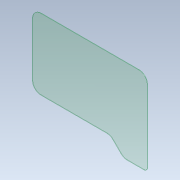
# Autodesk Inventor part: Стекло
Saved by Autodesk Inventor 2021.2 (Build 252289000, 289)
## iProperties
Created: 2022-11-29
Part Number: Стекло
Material: Типовые
Document SubType Name: ЛистМат
Designer: Voodoo
Density: 1 g/cm^3
Sheet Metal Rule: По умолчанию_мм
Appearance: Прозрачный — зеленый 1
Mass: 244.688 g
Surface Area: 2475.51 cm^2
Volume: 244.688 cm^3
Flat Pattern Width: 31.9 cm
Flat Pattern Length: 43.6 cm
Flat Pattern Area: 1390.84 cm^2
Sheet Metal Width: 319,000 мм
Sheet Metal Length: 436,000 мм
Sheet Metal Area: 139084,000 мм^2
Author: Voodoo
Autodesk Inventor part; units mm, degrees
ref_plane "YZ Plane" through (0, 0, 0) normal (1, 0, 0) x (0, 1, 0)
ref_plane "XZ Plane" through (0, 0, 0) normal (0, 1, 0) x (-1, 0, 0)
ref_plane "XY Plane" through (0, 0, 0) normal (0, 0, 1) x (1, 0, 0)
sketch "Эскиз1" plane through (0, 0, 0) normal (0, 0, 1) x (1, 0, 0)
  line L0 (-186, -134.5) -> (65.5736, -134.5)
  line L1 (218, -134.5) -> (218, 102.5)
  line L2 (186, 134.5) -> (-186, 134.5)
  line L3 (-218, 102.5) -> (-218, -102.5)
  line L4 (-218, -134.5) -> (218, 134.5) construction
  line L5 (218, -134.5) -> (-218, 134.5) construction
  arc A0 (-186, 134.5) -> (-218, 102.5) centre (-186, 102.5) ccw
  arc A1 (218, 102.5) -> (186, 134.5) centre (186, 102.5) ccw
  arc A2 (-218, -102.5) -> (-186, -134.5) centre (-186, -102.5) ccw
  line L6 (218, -134.5) -> (218, -172.5)
  line L7 (206, -184.5) -> (140.4264, -184.5)
  line L8 (119.2132, -175.7132) -> (86.7868, -143.2868)
  arc A3 (206, -184.5) -> (218, -172.5) centre (206, -172.5) ccw
  arc A4 (119.2132, -175.7132) -> (140.4264, -184.5) centre (140.4264, -154.5) ccw
  arc A5 (86.7868, -143.2868) -> (65.5736, -134.5) centre (65.5736, -164.5) ccw
  point P0 (0, 0)
  point P1 (218, -184.5)
  point P2 (128, -184.5)
  dimension "d2" = 436
  dimension "d3" = 269
  dimension "d4" = 32
  dimension "d5" = 319
  dimension "d6" = 12
  dimension "d7" = 50
  dimension "d8" = 90
  dimension "d9" = 135
  dimension "d10" = 30
  measures "d2" distance of L5.end L4.end
  measures "d3" distance of L4.end L1.start
  measures "d4" radius of A0
  measures "d5" distance between parallel lines of L7 L2
  measures "d6" radius of A3
  measures "d7" distance between parallel lines of L0 L7
  measures "d8" distance from line of L6 point (128, -184.5)
  measures "d9" angle of L0 L8
  measures "d10" radius of A4
extrude "Пластина1" add sketch "Эскиз1" along normal blind 2
equation "\"d12\" = Толщина"
equation "\"Радиус_гибки\" = Толщина"
equation "\"Ширина_просечки\" = Толщина"
equation "\"Глубина_просечки\" = 0.5 * Толщина"
equation "\"Размер_просечки\" = 4 * Толщина"
equation "\"Мин_остаток\" = 2 * Толщина"
equation "\"Радиус_перехода\" = Радиус_гибки"
equation "\"Радиус_Якоби\" = Радиус_гибки"
equation "\"Размер_зазора\" = Толщина"
equation "\"Толщина\" = 2"
